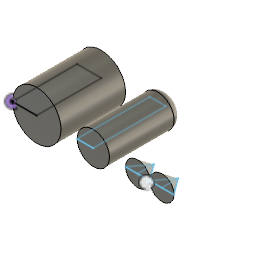
stud5 (Autodesk Fusion 360 design; units mm, degrees)
part number: 2025-12-06-14-40-35-873
Autodesk Fusion 360 part; units mm, degrees
sketch "스케치1" plane through (0, 0, 0) normal (0, 0, 1) x (1, 0, 0)
  line L0 (0, 0) -> (15, 0)
  line L1 (15, 0) -> (15, 40)
  line L2 (15, 40) -> (0, 40)
  line L3 (0, 40) -> (0, 0)
  line L4 (40, 0) -> (50, 0)
  line L5 (50, 0) -> (50, 45)
  line L6 (50, 45) -> (40, 45)
  line L7 (40, 45) -> (40, 0)
  line L8 (70, 0) -> (85, 0)
  line L9 (85, 0) -> (100, 0)
  line L10 (77.5, 0) -> (77.5, 10)
  line L11 (92.5, 0) -> (92.5, 10)
  line L12 (70, 0) -> (77.5, 10)
  line L13 (77.5, 10) -> (85, 0)
  line L14 (85, 0) -> (92.5, 10)
  line L15 (92.5, 10) -> (100, 0)
  line L16 (85, 0) -> (85, -2)
  dimension "d1" = 15
  dimension "d2" = 40
  dimension "d3" = 10
  dimension "d4" = 45
  dimension "d5" = 15
  dimension "d6" = 15
  constraint horizontal L0
  constraint vertical L1
  constraint horizontal L2
  constraint vertical L3
  constraint coincident L0.start L3.end
  constraint horizontal L4
  constraint vertical L5
  constraint horizontal L6
  constraint vertical L7
  constraint horizontal L8
  constraint perpendicular L3 L9
  constraint perpendicular L8 L10
  constraint perpendicular L9 L11
  constraint coincident L8 L10.start
  constraint coincident L9 L11.start
  constraint symmetric L10 L12 L13
  constraint symmetric L11 L14 L15
  constraint perpendicular L9 L16
  measures "d1" distance of L0.start L0.end
  measures "d2" distance of L0.start L2.end
  measures "d3" distance of L4.start L4.end
  measures "d4" distance of L4.start L6.end
  measures "d5" distance of L8.start L8.end
  measures "d6" distance of L8.end L9.end
revolve "회전1" add sketch "스케치1" angle 360 about axis through (15, 0, 0) along (0, 1, 0) contours L0 L1 L2 L3 makes body 1
revolve "회전2" add sketch "스케치1" angle 360 about axis through (50, 0, 0) along (0, 1, 0) separate body contours L4 L5 L6 L7 makes body 2
revolve "회전3" add sketch "스케치1" angle 360 about axis through (77.5, 0, 0) along (0, 1, 0) separate body contours L8 L10 L12 makes body 3
revolve "회전4" add sketch "스케치1" angle 360 about axis through (92.5, 0, 0) along (0, 1, 0) separate body contours L9 L11 L14 makes body 4
fillet "필렛1" radius 5 1 edges at (40.6767, 45, 3.6162) on bodies 2
